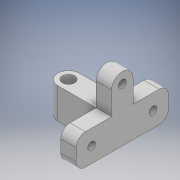
# Autodesk Inventor part: frame mount 1
Saved by Autodesk Inventor 2017 (Build 210142000, 142)
## iProperties
Created: 2017-12-13
Part Number: frame mount 1
Material: Generic
Document SubType Name: Modeling
Designer: RLanting
Density: 1 g/cm^3
Appearance: Default
Author: RLanting
Autodesk Inventor part; units mm, degrees
ref_plane "YZ Plane" through (0, 0, 0) normal (1, 0, 0) x (0, 1, 0)
ref_plane "XZ Plane" through (0, 0, 0) normal (0, 1, 0) x (-1, 0, 0)
ref_plane "XY Plane" through (0, 0, 0) normal (0, 0, 1) x (1, 0, 0)
sketch "Sketch1" plane through (0, 0, 0) normal (0, 0, 1) x (1, 0, 0)
  line L0 (0, 0) -> (-25, 0) construction
  circle A0 centre (-25, 0) radius 4
  line L1 (10, 30) -> (0, 30)
  line L2 (0, 30) -> (0, -30)
  line L3 (0, -30) -> (10, -30)
  line L4 (10, -30) -> (10, 30)
  line L5 (0, 0) -> (-25, 0) construction
  line L6 (0, 7) -> (-25, 7)
  line L7 (-25, -7) -> (0, -7)
  arc A1 (0, -7) -> (0, 7) centre (0, 0) ccw
  arc A2 (-25, 7) -> (-25, -7) centre (-25, 0) ccw
  point P0 (-12.5, 0)
  dimension "d0" = 8
  dimension "d1" = 25
  dimension "d2" = 60
  dimension "d3" = 10
  dimension "d4" = 7
  constraints: 18 end point, 4 equal length, 4 point on circle, 4 tangent, 3 centre point, 2 horizontal, 2 midpoint, 1 coincident, 1 perpendicular
  measures "d0" diameter of A0
  measures "d1" distance of L0.start L0.end
  measures "d2" distance of L1.end L2.end
  measures "d3" distance of L1.start L1.end
  measures "d4" radius of A2
extrude "Extrusion1" add sketch "Sketch1" along normal blind 20
sketch "Sketch2" plane through (10, -30, 0) normal (1, 0, 0) x (0, 0, -1)
  line L0 (0, 60) -> (-20, 60) construction
  line L1 (-10, 60) -> (-10, 50) construction
  line L2 (0, 0) -> (-20, 0) construction
  line L3 (-10, 0) -> (-10, 10) construction
  circle A0 centre (-10, 50) radius 2.5
  circle A1 centre (-10, 10) radius 2.5
  point P0 (0, 30)
  dimension "d7" = 5
  dimension "d8" = 10
  constraints: 4 end point, 2 centre point, 2 coincident, 2 midpoint, 2 vertical, 1 collinear, 1 equal radius
  measures "d7" diameter of A1
  measures "d8" distance of L3.start L3.end
extrude "Extrusion2" cut sketch "Sketch2" against normal through all
fillet "Fillet1" radius 6 4 edges at (5, 30, 20) (5, 30, 0) (5, -30, 20) (5, -30, 0)
sketch "Sketch3" plane through (10, -24, 0) normal (1, 0, 0) x (0, 0, -1)
  line L0 (-20, 20) -> (-20, 28) projected
  line L1 (-20, 24) -> (-35, 24) construction
  line L2 (-20, 31) -> (-35, 31)
  line L3 (-35, 17) -> (-20, 17)
  arc A0 (-20, 17) -> (-20, 31) centre (-20, 24) ccw
  arc A1 (-35, 31) -> (-35, 17) centre (-35, 24) ccw
  circle A2 centre (-35, 24) radius 2.5
  point P0 (0, 24)
  point P1 (-27.5, 24)
  dimension "d12" = 5
  dimension "d13" = 7
  dimension "d14" = 15
  constraints: 8 end point, 4 point on circle, 4 tangent, 3 centre point, 2 midpoint, 1 coincident, 1 horizontal, 1 parallel
  measures "d12" diameter of A2
  measures "d13" radius of A1
  measures "d14" distance of L1.start L1.end
extrude "Extrusion3" add sketch "Sketch3" against normal blind 10
body "Solid1"
